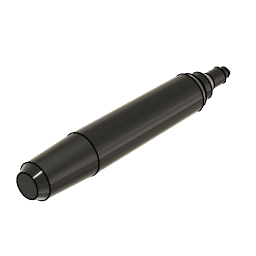
Marcador (Autodesk Fusion 360 design; units mm, degrees)
Autodesk Fusion 360 part; units mm, degrees
sketch "Boceto2" plane through (0, 0, 0) normal (0, 1, 0) x (1, 0, 0)
  circle A0 centre (0, 0) radius 6.6
  dimension "d1" = 13.2
  constraint coincident A0.centre origin
  measures "d1" diameter of A0
ref_plane "PlanoDeObra1" through (0, 5, 0) normal (0, 1, 0) x (1, 0, 0)
sketch "Boceto3" plane through (0, 5, 0) normal (0, 1, 0) x (1, 0, 0)
  circle A0 centre (0, 0) radius 9.4
  dimension "d3" = 18.8
  constraint coincident A0.centre origin
  measures "d3" diameter of A0
ref_plane "PlanoDeObra2" through (0, 34.5, 0) normal (0, 1, 0) x (1, 0, 0)
sketch "Boceto4" plane through (0, 34.5, 0) normal (0, 1, 0) x (1, 0, 0)
  circle A0 centre (0, 0) radius 10.65
  dimension "d5" = 21.3
  constraint coincident A0.centre origin
  measures "d5" diameter of A0
loft "Solevación1" add profiles "Boceto2", "Boceto3" section 1 section 2
loft "Solevación2" add profiles "Boceto4" section 1 face at (2.1836, 5, -0.9236) section 2
ref_plane "PlanoDeObra3" through (0, 101.7, 0) normal (0, 1, 0) x (0, 0, 1)
sketch "Boceto5" plane through (0, 101.7, 0) normal (0, 1, 0) x (1, 0, 0)
  circle A0 centre (0, 0) radius 9.25
  dimension "d7" = 18.5
  constraint coincident A0.centre origin
  measures "d7" diameter of A0
loft "Solevación3" add profiles "Boceto5" section 1 face at (-2.6023, 34.5, 4.1946) section 2
ref_plane "PlanoDeObra4" through (0, 104.5, 0) normal (0, 1, 0) x (0, 0, 1)
sketch "Boceto6" plane through (0, 104.5, 0) normal (0, 1, 0) x (1, 0, 0)
  circle A0 centre (0, 0) radius 8.15
  dimension "d9" = 16.3
  constraint coincident A0.centre origin
  measures "d9" diameter of A0
ref_plane "PlanoDeObra5" through (0, 109.7, 0) normal (0, 1, 0) x (1, 0, 0)
sketch "Boceto7" plane through (0, 109.7, 0) normal (0, 1, 0) x (1, 0, 0)
  circle A0 centre (0, 0) radius 6.55
  dimension "d11" = 13.1
  constraint coincident A0.centre origin
  measures "d11" diameter of A0
ref_plane "PlanoDeObra6" through (0, 120.9, 0) normal (0, 1, 0) x (1, 0, 0)
sketch "Boceto8" plane through (0, 120.9, 0) normal (0, 1, 0) x (1, 0, 0)
  circle A0 centre (0, 0) radius 4
  dimension "d13" = 8
  constraint coincident A0.centre origin
  measures "d13" diameter of A0
loft "Solevación4" add profiles "Boceto6" section 1 face at (-2.5312, 101.7, -3.8946) section 2
extrude "Extruir1" add sketch "Boceto7" against normal blind 5.2
extrude "Extruir2" add sketch "Boceto8" against normal blind 11.2
fillet "Empalme1" radius 1.5 1 edges at (-6.1067, 104.5, -2.3686)
chamfer "Chaflán1" distance 2.55 distance2 4 1 edges at (-3.7293, 109.7, -1.4465) measured on face at (5.6756, 109.7, 0.3254)
ref_plane "PlanoDeObra7" through (0, 126.7, 0) normal (0, -1, 0) x (0, 0, -1)
sketch "Boceto9" plane through (0, 120.9, 0) normal (0, 1, 0) x (-1, 0, 0)
  circle A0 centre (0, 0) radius 4
  circle A1 centre (0, 0) radius 2.6
  dimension "d23" = 5.2
  constraint concentric A0 A1
  measures "d23" diameter of A1
extrude "Extruir3" add sketch "Boceto9" along normal up to surface (5.8 mm away) contours A1
fillet "Empalme2" radius 2.47 tangency weight 0.5 1 edges at (2.4241, 126.7, -0.9402)
equation "d4 = 25.5 mm + 4 mm"
equation "d27 = ( ( 5.2 / 2 ) * 0.95 ) * 1 mm"
